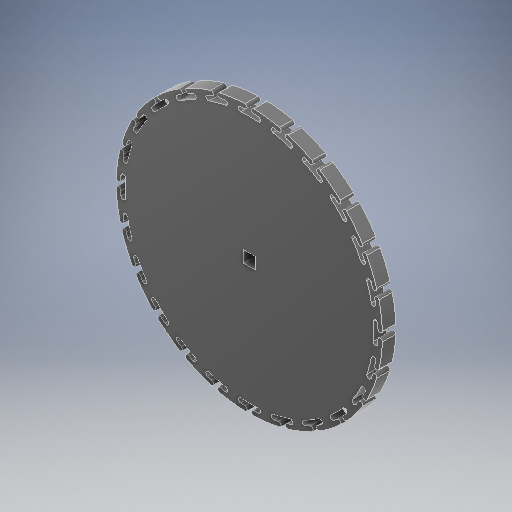
# Autodesk Inventor part: Custom-Roller-LS
Saved by Autodesk Inventor 2026.1 (Build 301233000, 233)
## iProperties
Created: 2025-10-16
Part Number: Custom-Roller-LS
Material: Plastic, Opaque Black
Document SubType Name: Modeling
Designer: Teddy
Density: 0.952 g/cm^3
Appearance: Smooth - Black
Diam: 3.000 in
HighStength: False
Author: Teddy
Autodesk Inventor part; units mm, degrees
ref_plane "YZ Plane" through (0, 0, 0) normal (1, 0, 0) x (0, 1, 0)
ref_plane "XZ Plane" through (0, 0, 0) normal (0, 1, 0) x (-1, 0, 0)
ref_plane "XY Plane" through (0, 0, 0) normal (0, 0, 1) x (1, 0, 0)
sketch "Sketch1" plane through (0, 0, 0) normal (0, 0, 1) x (1, 0, 0)
  circle A0 centre (0, 0) radius 38.1
  line L0 (-1.651, -1.651) -> (1.651, -1.651)
  line L1 (1.651, -1.651) -> (1.651, 1.651)
  line L2 (1.651, 1.651) -> (-1.651, 1.651)
  line L3 (-1.651, 1.651) -> (-1.651, -1.651)
  line L4 (-1.651, -1.651) -> (1.651, 1.651) construction
  line L5 (1.651, -1.651) -> (-1.651, 1.651) construction
  dimension "Diam_Sketch" = 76.2
  dimension "LowStrengthWidth" = 3.302
  constraints: 12 end point, 2 midpoint, 2 parallel, 2 perpendicular, 1 centre point, 1 coincident, 1 horizontal
  measures "Diam_Sketch" diameter of A0
  measures "LowStrengthWidth" distance of L1.end L2.end
extrude "Extrusion1" add sketch "Sketch1" along normal blind 3.81
sketch "Sketch2" plane through (0, 0, 3.81) normal (0, 0, 1) x (1, 0, 0)
  line L0 (-3.302, -3.302) -> (3.302, -3.302)
  line L1 (3.302, -3.302) -> (3.302, 3.302)
  line L2 (3.302, 3.302) -> (-3.302, 3.302)
  line L3 (-3.302, 3.302) -> (-3.302, -3.302)
  line L4 (-3.302, -3.302) -> (3.302, 3.302) construction
  line L5 (3.302, -3.302) -> (-3.302, 3.302) construction
  point P0 (0, 0)
  dimension "HighStrengthWidth" = 6.604
  constraints: 12 end point, 2 midpoint, 2 parallel, 2 perpendicular, 1 horizontal
  measures "HighStrengthWidth" distance of L1.end L2.end
extrude "HighStrenthCut" [suppressed]
sketch "Sketch3" plane through (0, 0, 3.81) normal (0, 0, 1) x (1, 0, 0)
  circle A0 centre (0, 0) radius 36.195 construction
  arc A1 (2.54, 36.1058) -> (-2.54, 36.1058) centre (0, 0) ccw construction
  arc A2 (2.5846, 36.7392) -> (-2.5846, 36.7392) centre (0, 0) ccw
  arc A3 (2.4954, 35.4723) -> (-2.4954, 35.4723) centre (0, 0) ccw
  arc A4 (2.4954, 35.4723) -> (2.5846, 36.7392) centre (2.54, 36.1058) ccw
  arc A5 (-2.5846, 36.7392) -> (-2.4954, 35.4723) centre (-2.54, 36.1058) ccw
  line L0 (-2.54, 36.1058) -> (0, 0) construction
  line L1 (0, 0) -> (2.54, 36.1058) construction
  line L2 (0, 0) -> (0, 36.195) construction
  arc A6 (-1.2485, 36.8088) -> (-1.2915, 38.0781) centre (-1.27, 37.4435) ccw
  arc A7 (1.2915, 38.0781) -> (1.2485, 36.8088) centre (1.27, 37.4435) ccw
  circle A8 centre (0, 0) radius 38.1 projected
  arc A9 (-1.3134, 39.37) -> (-1.2915, 38.0781) centre (-1.3134, 38.7239) ccw
  line L3 (-1.3134, 39.37) -> (1.3134, 39.37)
  arc A10 (1.2915, 38.0781) -> (1.3134, 39.37) centre (1.3134, 38.7239) ccw
  dimension "ToothDiam" = 72.39
  dimension "ToothLength" = 5.08
  dimension "ToothWidth" = 1.27
  dimension "OutsideCut" = 39.37
  constraints: 21 point on circle, 13 tangent, 9 centre point, 8 end point, 2 coincident, 1 equal radius, 1 horizontal, 1 symmetric about line, 1 vertical, 5 other
  measures "ToothLength" distance of L1.end L0.start
  measures "OutsideCut" distance from line of A8.centre L3
extrude "Extrusion3" cut sketch "Sketch3" against normal blind 3.81 contours A4 A3 A5 A2 | A2 A6 A8 A7 | A8 A9 L3 A10
pattern_circular "Circular Pattern1" count 24 over 360 about axis through (0, 0, 0) along (0, 0, 1) of "Extrusion3"
equation "\"Diam_Sketch\" = Diam"
equation "\"HighStrengthCutDepth\" = SprocketWidth"
equation "\"ToothDepth\" = SprocketWidth"
equation "\"Diam\" = 76.2"
equation "\"SprocketWidth\" = 3.81"
body "Solid1"
